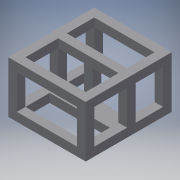
# Autodesk Inventor part: BSF_OuterFrame
Saved by Autodesk Inventor 2018 (Build 220112000, 112)
## iProperties
Created: 2019-03-24
Part Number: BSF_OuterFrame
Material: Generic
Document SubType Name: Modeling
Designer: simon
Density: 1 g/cm^3
Appearance: Default
Author: simon
Autodesk Inventor part; units mm, degrees
ref_plane "YZ Plane" through (0, 0, 0) normal (1, 0, 0) x (0, 1, 0)
ref_plane "XZ Plane" through (0, 0, 0) normal (0, 1, 0) x (-1, 0, 0)
ref_plane "XY Plane" through (0, 0, 0) normal (0, 0, 1) x (1, 0, 0)
sketch "Sketch1" plane through (0, 0, 0) normal (0, 0, 1) x (1, 0, 0)
  line L0 (250, 0) -> (0, 0) projected
  line L1 (250, 0) -> (250, 40) projected
  line L2 (211.5, 40) -> (250, 40) projected
  line L3 (161.5, 40) -> (211.5, 40) projected
  line L4 (88.5, 40) -> (161.5, 40) projected
  line L5 (38.5, 40) -> (88.5, 40) projected
  line L6 (0, 40) -> (38.5, 40) projected
  line L7 (0, 0) -> (0, 40) projected
  line L8 (-15, 40) -> (-55, 40)
  line L9 (-55, 40) -> (-55, -360)
  line L10 (-55, -360) -> (-15, -360)
  line L11 (-15, -360) -> (-15, 40)
  line L12 (265, 40) -> (305, 40)
  line L13 (305, 40) -> (305, -360)
  line L14 (305, -360) -> (265, -360)
  line L15 (265, -360) -> (265, 40)
  line L16 (265, -360) -> (-15, -360)
  line L17 (-15, -360) -> (-15, -320)
  line L18 (-15, -320) -> (265, -320)
  line L19 (265, -320) -> (265, -360)
  line L20 (265, -127.6607) -> (-15, -127.6607)
  line L21 (-15, -127.6607) -> (-15, -207.6607)
  line L22 (-15, -207.6607) -> (265, -207.6607)
  line L23 (265, -207.6607) -> (265, -127.6607)
  dimension "d0" = 40
  dimension "d1" = 400
  dimension "d2" = 40
  dimension "d3" = 400
  dimension "d4" = 15
  dimension "d5" = 15
  dimension "d6" = 40
  dimension "d9" = 80
  constraints: 32 end point, 8 parallel, 4 horizontal, 4 perpendicular, 4 point on line
  measures "d0" distance of L10.end L9.end
  measures "d1" distance of L9.end L8.end
  measures "d2" distance of L13.end L14.end
  measures "d3" distance of L12.end L13.end
  measures "d4" distance between parallel lines of L15 L1
  measures "d5" distance between parallel lines of L7 L11
  measures "d6" distance of L16.end L17.end
  measures "d9" distance of L21.end L20.end
extrude "Extrusion1" add sketch "Sketch1" against normal blind 40 contours L11 L10 L9 L8 | L20 L15 L22 L11 | L15 L12 L13 L14 | L11 L18 L15 L16
sketch "Sketch2" plane through (0, 0, -40) normal (0, 0, -1) x (-1, 0, 0)
  line L0 (-265, -207.6607) -> (15, -207.6607) projected
  line L1 (15, -207.6607) -> (15, -320) projected
  line L2 (15, -320) -> (-265, -320) projected
  line L3 (-265, -320) -> (-265, -207.6607) projected
  line L4 (-265, -127.6607) -> (-265, 40) projected
  line L5 (-265, 40) -> (-305, 40) projected
  line L6 (-305, 40) -> (-305, -360) projected
  line L7 (-305, -360) -> (55, -360) projected
  line L8 (55, -360) -> (55, 40) projected
  line L9 (55, 40) -> (15, 40) projected
  line L10 (15, 40) -> (15, -127.6607) projected
  line L11 (15, -127.6607) -> (-265, -127.6607) projected
  line L12 (-103, -127.6607) -> (-147, -127.6607)
  line L13 (-147, -127.6607) -> (-147, -83.6607)
  line L14 (-147, -83.6607) -> (-103, -83.6607)
  line L15 (-103, -83.6607) -> (-103, -127.6607)
  point P0 (0, 0)
  dimension "d10" = 44
  dimension "d11" = 44
  dimension "d12" = 118
  dimension "d13" = 118
  constraints: 8 end point, 2 parallel, 1 horizontal, 1 perpendicular, 1 point on line
  measures "d10" distance of L13.end L14.end
  measures "d11" distance of L12.end L13.end
  measures "d12" distance between parallel lines of L10 L15
  measures "d13" distance between parallel lines of L4 L13
extrude "Extrusion2" add sketch "Sketch2" along normal blind 44 contours L13 L14 L15 L11
sketch "Sketch3" plane through (0, 0, -40) normal (0, 0, 1) x (1, 0, 0)
  line L0 (103, -127.6607) -> (103, -83.6607) projected
  line L1 (103, -127.6607) -> (147, -127.6607) projected
  line L2 (147, -83.6607) -> (147, -127.6607) projected
  line L3 (103, -83.6607) -> (147, -83.6607) projected
  circle A0 centre (125, -105.6607) radius 2.5
  point P0 (0, 0)
  dimension "d16" = 5
  constraints: 1 centre point
  measures "d16" diameter of A0
extrude "Extrusion3" add sketch "Sketch3" along normal blind 20 contours A0
sketch "Sketch4" plane through (0, 0, 0) normal (0, 0, 1) x (1, 0, 0)
  line L0 (147, -127.6607) -> (265, -127.6607) projected
  line L1 (103, -127.6607) -> (147, -127.6607) projected
  line L2 (125, -127.6607) -> (125, -147.6607)
  line L3 (105, -127.6607) -> (145, -127.6607)
  line L4 (145, -127.6607) -> (145, -167.6607)
  line L5 (145, -167.6607) -> (105, -167.6607)
  line L6 (105, -167.6607) -> (105, -127.6607)
  line L7 (105, -127.6607) -> (145, -167.6607) construction
  line L8 (145, -127.6607) -> (105, -167.6607) construction
  line L9 (305, -360) -> (-55, -360) projected
  line L10 (-15, -320) -> (265, -320) projected
  line L11 (305, -360) -> (265, -360)
  line L12 (265, -360) -> (265, -320)
  line L13 (265, -320) -> (305, -320)
  line L14 (305, -320) -> (305, -360)
  line L15 (-15, -207.6607) -> (-15, -320) projected
  line L16 (-55, -360) -> (-15, -360)
  line L17 (-15, -360) -> (-15, -320)
  line L18 (-15, -320) -> (-55, -320)
  line L19 (-55, -320) -> (-55, -360)
  line L20 (305, -360) -> (305, 40) projected
  line L21 (265, -127.6607) -> (305, -127.6607)
  line L22 (305, -127.6607) -> (305, -167.6607)
  line L23 (305, -167.6607) -> (265, -167.6607)
  line L24 (265, -167.6607) -> (265, -127.6607)
  line L25 (-15, 40) -> (-15, -127.6607) projected
  line L26 (-55, -360) -> (-55, 40) projected
  line L27 (-15, -127.6607) -> (-55, -127.6607)
  line L28 (-55, -127.6607) -> (-55, -167.6607)
  line L29 (-55, -167.6607) -> (-15, -167.6607)
  line L30 (-15, -167.6607) -> (-15, -127.6607)
  line L31 (305, 40) -> (265, 40)
  line L32 (265, 40) -> (265, 0)
  line L33 (265, 0) -> (305, 0)
  line L34 (305, 0) -> (305, 40)
  line L35 (-55, 40) -> (-15, 40)
  line L36 (-15, 40) -> (-15, 0)
  line L37 (-15, 0) -> (-55, 0)
  line L38 (-55, 0) -> (-55, 40)
  point P0 (0, 0)
  dimension "d21" = 20
  dimension "d22" = 40
  dimension "d23" = 40
  dimension "d28" = 40
  dimension "d29" = 40
  dimension "d30" = 40
  dimension "d31" = 40
  constraints: 62 end point, 14 parallel, 7 horizontal, 7 perpendicular, 3 midpoint, 3 point on line, 1 vertical
  measures "d21" distance of L2.start L2.end
  measures "d22" distance of L4.end L5.end
  measures "d23" distance of L3.end L4.end
  measures "d28" distance of L33.end L32.end
  measures "d29" distance of L32.end L31.end
  measures "d30" distance of L36.end L37.end
  measures "d31" distance of L35.end L36.end
extrude "Extrusion4" add sketch "Sketch4" along normal blind 200 contours L33 L32 L31 L20 | L26 L27 L30 L29 | L14 L9 L12 L13 | L21 L20 L23 L24 | L4 L5 L6 L1 | L17 L9 L19 L18 | L26 L35 L25 L37
sketch "Sketch5" plane through (0, 0, 200) normal (0, 0, 1) x (1, 0, 0)
  line L0 (265, -167.6607) -> (305, -167.6607) projected
  line L1 (305, -360) -> (305, -320) projected
  line L2 (265, -167.6607) -> (305, -167.6607)
  line L3 (305, -167.6607) -> (305, -320)
  line L4 (305, -320) -> (265, -320)
  line L5 (265, -320) -> (265, -167.6607)
  line L6 (265, -167.6607) -> (145, -167.6607)
  line L7 (145, -167.6607) -> (145, -127.6607)
  line L8 (145, -127.6607) -> (265, -127.6607)
  line L9 (265, -127.6607) -> (265, -167.6607)
  line L10 (105, -167.6607) -> (145, -167.6607) projected
  line L11 (105, -167.6607) -> (-15, -167.6607)
  line L12 (-15, -167.6607) -> (-15, -127.6607)
  line L13 (-15, -127.6607) -> (105, -127.6607)
  line L14 (105, -127.6607) -> (105, -167.6607)
  line L15 (-55, -127.6607) -> (-55, -167.6607) projected
  line L16 (-55, -167.6607) -> (-15, -167.6607)
  line L17 (-15, -167.6607) -> (-15, -320)
  line L18 (-15, -320) -> (-55, -320)
  line L19 (-55, -320) -> (-55, -167.6607)
  line L20 (-15, -320) -> (265, -320)
  line L21 (265, -320) -> (265, -360)
  line L22 (265, -360) -> (-15, -360)
  line L23 (-15, -360) -> (-15, -320)
  line L24 (305, -167.6607) -> (305, -127.6607) projected
  line L25 (265, 40) -> (265, 0) projected
  line L26 (305, -127.6607) -> (265, -127.6607)
  line L27 (265, -127.6607) -> (265, 0)
  line L28 (265, 0) -> (305, 0)
  line L29 (305, 0) -> (305, -127.6607)
  line L30 (265, 40) -> (-15, 40)
  line L31 (-15, 40) -> (-15, 0)
  line L32 (-15, 0) -> (265, 0)
  line L33 (265, 0) -> (265, 40)
  line L34 (-15, 0) -> (-55, 0)
  line L35 (-55, 0) -> (-55, -127.6607)
  line L36 (-55, -127.6607) -> (-15, -127.6607)
  line L37 (-15, -127.6607) -> (-15, 0)
  point P0 (0, 0)
  constraints: 64 end point, 16 parallel, 8 horizontal, 8 perpendicular
extrude "Extrusion5" add sketch "Sketch5" against normal blind 40 contours L0 L3 L4 L5 | L6 L7 L8 L9 | L21 L22 L23 L20 | L27 L28 L29 L26 | L18 L19 L16 L17 | L11 L12 L13 L14 | L32 L31 L30 L25 | L37 L36 L35 L34
body "Solid1"
